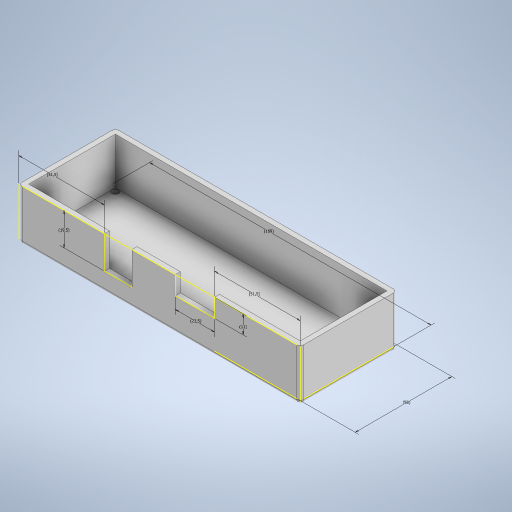
# Autodesk Inventor part: Part1
Saved by Autodesk Inventor 2024 (Build 280153000, 153)
## iProperties
Created: 2025-02-27
Part Number: Part1
Material: Generic
Document SubType Name: Modeling
Designer: vandevelde.wout
Density: 1 g/cm^3
Appearance: Default
Author: vandevelde.wout
Autodesk Inventor part; units mm, degrees
ref_plane "YZ Plane" through (0, 0, 0) normal (1, 0, 0) x (0, 1, 0)
ref_plane "XZ Plane" through (0, 0, 0) normal (0, 1, 0) x (-1, 0, 0)
ref_plane "XY Plane" through (0, 0, 0) normal (0, 0, 1) x (1, 0, 0)
sketch "Sketch1" plane through (0, 0, 0) normal (0, 1, 0) x (-1, 0, 0)
  line L0 (0, 0) -> (163, 0)
  line L1 (163, 0) -> (163, -52)
  line L2 (163, -52) -> (0, -52)
  line L3 (0, -52) -> (0, 0)
  line L4 (0, 0) -> (-3, 0)
  line L5 (-3, 0) -> (-3, 3)
  line L6 (-3, 3) -> (166, 3)
  line L7 (166, 3) -> (166, -55)
  line L8 (166, -55) -> (-3, -55)
  line L9 (-3, 0) -> (-3, -55)
  dimension "d0" = 163
  dimension "d1" = 52
  dimension "d2" = 3
  dimension "d3" = 3
  dimension "d4" = 169
  dimension "d5" = 58
  dimension "d6" = 169
  constraints: 20 end point, 4 perpendicular, 2 horizontal, 2 parallel, 1 vertical
  measures "d0" distance of L1.end L2.end
  measures "d1" distance of L0.end L1.end
  measures "d2" distance of L0.start L4.end
  measures "d3" distance of L4.end L5.end
  measures "d4" distance of L5.end L6.end
  measures "d5" distance of L6.end L7.end
  measures "d6" distance of L7.end L8.end
extrude "Extrusion1" add sketch "Sketch1" along normal blind 28
sketch "Sketch2" plane through (-166, 0, 3) normal (0, 0, 1) x (1, 0, 0)
  line L0 (169, 0) -> (0, 0) projected
  line L1 (0, 0) -> (169, 0)
  line L2 (169, 0) -> (169, -2.5)
  line L3 (169, -2.5) -> (0, -2.5)
  line L4 (0, -2.5) -> (0, 0)
  point P0 (166, 0)
  dimension "d9" = 2.5
  constraints: 8 end point, 2 parallel, 1 horizontal, 1 perpendicular
  measures "d9" distance of L1.end L2.end
extrude "Extrusion2" add sketch "Sketch2" against normal blind 58
sketch "Sketch3" plane through (-166, 28, 3) normal (0, 0, 1) x (1, 0, 0)
  line L0 (94, 0) -> (117.5, 0)
  line L1 (117.5, 0) -> (117.5, -11)
  line L2 (117.5, -11) -> (94, -11)
  line L3 (94, -11) -> (94, 0)
  line L4 (169, -30.5) -> (169, 0) projected
  line L5 (0, -30.5) -> (0, 0) projected
  line L6 (166, -28) -> (3, -28) projected
  line L7 (0, 0) -> (169, 0) projected
  line L8 (51.5, -11) -> (68, -11)
  line L9 (68, -11) -> (68, -19.5)
  line L10 (68, -19.5) -> (51.5, -19.5)
  line L11 (51.5, -19.5) -> (51.5, -11)
  line L12 (51.5, -11) -> (68, -19.5) construction
  line L13 (68, -11) -> (51.5, -19.5) construction
  line L14 (0, -30.5) -> (169, -30.5) projected
  line L15 (51.5, -11) -> (51.5, 0)
  line L16 (68, -11) -> (68, 0)
  line L17 (51.5, 0) -> (68, 0)
  point P0 (59.75, -15.25)
  dimension "d12" = 75
  dimension "d13" = 117.5
  dimension "d14" = 17
  dimension "d15" = 0
  dimension "d16" = 23.5
  dimension "d17" = 16.5
  dimension "d18" = 8.5
  dimension "d19" = 30.5
  dimension "d20" = 15.25
  dimension "d21" = 51.5
  dimension "d22" = 51.5
  constraints: 26 end point, 4 parallel, 4 perpendicular, 2 horizontal, 2 midpoint, 2 point on line, 1 collinear
  measures "d12" distance between parallel lines of L4 L3
  measures "d13" distance between parallel lines of L5 L1
  measures "d14" distance between parallel lines of L2 L6
  measures "d15" distance between parallel lines of L7 L0
  measures "d16" distance between parallel lines of L1 L3
  measures "d17" distance between parallel lines of L9 L11
  measures "d18" distance between parallel lines of L8 L10
  measures "d19" distance between parallel lines of L14 L7
  measures "d20" distance from line of L7 point (59.75, -15.25)
  measures "d21" distance between parallel lines of L4 L1
  measures "d22" distance between parallel lines of L5 L11
extrude "Extrusion3" cut sketch "Sketch3" against normal blind 10 contours L0 L1 L2 L3 | L16 L8 L15 L7 | L9 L10 L11 L8
sketch "Sketch4" plane through (-166, -2.5, 3) normal (0, 0, 1) x (1, 0, 0)
  point P0 (166, 2.5)
sketch "Sketch5" plane through (-163, 0, -52) normal (0, 1, 0) x (1, 0, 0)
  circle A0 centre (161, -50) radius 2
  circle A1 centre (161, -2) radius 2
  circle A2 centre (2, -2) radius 2
  circle A3 centre (2, -50) radius 2
  point P0 (163, -52)
  dimension "d25" = 4
  dimension "d26" = 4
  dimension "d27" = 4
  dimension "d28" = 4
  dimension "d29" = 48
  dimension "d30" = 159
  constraints: 4 centre point
  measures "d25" diameter of A0
  measures "d26" diameter of A1
  measures "d27" diameter of A2
  measures "d28" diameter of A3
  measures "d29" distance of A3.centre A2.centre
  measures "d30" distance of A0.centre A3.centre
extrude "Extrusion4" cut sketch "Sketch5" against normal blind 10
fillet "Fillet1" radius 2 8 edges at (3, 12.75, 3) (3, 12.75, -55) (-166, 12.75, -55) (-166, 12.75, 3) (-81.5, -2.5, -55) (-166, -2.5, -26) (-81.5, -2.5, 3) (3, -2.5, -26)
sketch "Sketch6" plane through (-161, 0, -52) normal (0, 1, 0) x (1, 0, 0)
  line L0 (164, -53) -> (164, 1) projected
  line L1 (-5, 1) -> (-5, -53) projected
  line L2 (162, 3) -> (-3, 3) projected
  line L3 (112.5, -55) -> (162, -55) projected
  point P0 (161, -52)
  dimension "d34" = 169
  dimension "d35" = 58
  measures "d34" distance between parallel lines of L0 L1
  measures "d35" distance between parallel lines of L2 L3
sketch "Sketch7" plane through (-98, 28, 3) normal (0, 0, 1) x (1, 0, 0)
  line L0 (49.5, 0) -> (49.5, -11) projected
  line L1 (101, -28.5) -> (101, 0) projected
  line L2 (26, -11) -> (49.5, -11) projected
  line L3 (99, 0) -> (-66, 0) projected
  line L4 (-68, 0) -> (-68, -28.5) projected
  line L5 (-16.5, -19.5) -> (-16.5, 0) projected
  line L6 (0, -19.5) -> (-16.5, -19.5) projected
  line L7 (26, -11) -> (26, 0) projected
  point P0 (98, -28)
  dimension "d36" = 51.5
  dimension "d37" = 11
  dimension "d38" = 51.5
  dimension "d39" = 19.5
  dimension "d40" = 23.5
  measures "d36" distance between parallel lines of L0 L1
  measures "d37" distance between parallel lines of L2 L3
  measures "d38" distance between parallel lines of L4 L5
  measures "d39" distance between parallel lines of L3 L6
  measures "d40" distance between parallel lines of L0 L7
body "Solid1"
